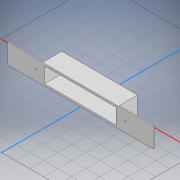
# Autodesk Inventor part: 000.009 - Короб
Saved by Autodesk Inventor 2022 (Build 260153000, 153)
## iProperties
Created: 2023-03-07
Part Number: 000.009 - Короб
Material: Типовые
Document SubType Name: Modeling
Designer: Иван Петров
Density: 1 g/cm^3
Appearance: По умолчанию
Author: Иван Петров
Autodesk Inventor part; units mm, degrees
ref_plane "YZ Plane" through (0, 0, 0) normal (1, 0, 0) x (0, 1, 0)
ref_plane "XZ Plane" through (0, 0, 0) normal (0, 1, 0) x (-1, 0, 0)
ref_plane "XY Plane" through (0, 0, 0) normal (0, 0, 1) x (1, 0, 0)
sketch "Эскиз1" plane through (0, 0, 0) normal (0, 0, 1) x (1, 0, 0)
  line L0 (-54, -14) -> (54, -14)
  line L1 (54, -14) -> (54, 14)
  line L2 (54, 14) -> (-54, 14)
  line L3 (-54, 14) -> (-54, -14)
  line L4 (-54, -14) -> (54, 14) construction
  line L5 (54, -14) -> (-54, 14) construction
  point P0 (0, 0)
  dimension "d0" = 108
  dimension "d1" = 28
  constraints: 12 end point, 2 midpoint, 2 parallel, 1 horizontal, 1 perpendicular
  measures "d0" distance of L2.end L1.end
  measures "d1" distance between parallel lines of L0 L2
extrude "Выдавливание1" add sketch "Эскиз1" along normal blind 27.5
sketch "Эскиз2" plane through (0, 0, 27.5) normal (0, 0, 1) x (1, 0, 0)
  line L0 (-51, -11) -> (51, -11)
  line L1 (51, -11) -> (51, 11)
  line L2 (51, 11) -> (-51, 11)
  line L3 (-51, 11) -> (-51, -11)
  line L4 (-51, -11) -> (51, 11) construction
  line L5 (51, -11) -> (-51, 11) construction
  line L6 (54, 14) -> (-54, 14) projected
  line L7 (54, -14) -> (54, 14) projected
  point P0 (0, 0)
  dimension "d4" = 3
  dimension "d5" = 3
  constraints: 12 end point, 2 midpoint, 2 parallel, 1 horizontal, 1 perpendicular
  measures "d4" distance between parallel lines of L6 L2
  measures "d5" distance between parallel lines of L7 L1
extrude "Выдавливание2" cut sketch "Эскиз2" against normal blind 24.5
sketch "Эскиз3" plane through (54, -14, 0) normal (1, 0, 0) x (0, 0, -1)
  line L0 (0, 28) -> (-27.5, 28) projected
  line L1 (0, 0) -> (-27.5, 0) projected
  line L2 (-27.5, 28) -> (-26, 28)
  line L3 (-26, 28) -> (-26, 0)
  line L4 (-26, 0) -> (-27.5, 0)
  line L5 (-27.5, 0) -> (-27.5, 28)
  point P0 (0, 14)
  dimension "d8" = 1.5
  constraints: 8 end point, 2 parallel, 1 horizontal, 1 perpendicular, 1 point on line
  measures "d8" distance between parallel lines of L5 L3
extrude "Выдавливание3" add sketch "Эскиз3" along normal blind 50
sketch "Эскиз4" plane through (0, 0, 27.5) normal (0, 0, 1) x (1, 0, 0)
  circle A0 centre (64, 0) radius 1.5
  line L0 (-54, -14) -> (104, -14) projected
  point P0 (0, 0)
  point P1 (54, -14)
  dimension "d11" = 3
  dimension "d12" = 14
  dimension "d13" = 10
  constraints: 1 centre point
  measures "d11" diameter of A0
  measures "d12" distance from line of L0 A0.centre
  measures "d13" horizontal distance of A0.centre point (54, -14)
extrude "Выдавливание4" cut sketch "Эскиз4" against normal blind 50
mirror "Зеркальное отражение1" about plane through (0, 0, 0) normal (1, 0, 0) of "Выдавливание3", "Выдавливание4"
